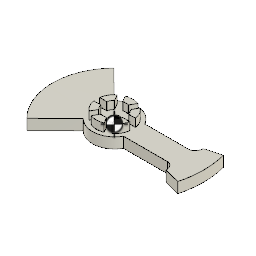
Hammer v2 v7 (Autodesk Fusion 360 design; units mm, degrees)
Autodesk Fusion 360 part; units mm, degrees
sketch "Sketch1" plane through (0, 0, 0) normal (0, 0, 1) x (1, 0, 0)
  circle A0 centre (0, 0) radius 2.7
  circle A1 centre (0, 0) radius 50
  line L0 (0, 0) -> (50, 0) construction
  line L1 (0, -6) -> (49.6387, -6)
  line L2 (0, 0) -> (48.3169, -12.864)
  spline S0 degree 5 poles (39.3956, -10.4888) (39.4086, -10.3289) (39.4175, -10.0126) (39.3796, -9.5486) (39.2342, -8.9536) (38.9326, -8.2648) (38.5571, -7.6509) (38.1484, -7.1313) (37.7328, -6.7198) (37.3076, -6.4144) (36.8464, -6.2013) (36.4204, -6.091) (36.0539, -6.0356) (35.7867, -6.01) (35.6473, -6) knots 0 0 0 0 0 0 0.1 0.2 0.3 0.4 0.5 0.6 0.7 0.8 0.9 1 1 1 1 1 1
  spline S1 degree 5 poles (39.3956, 10.4888) (39.4086, 10.3289) (39.4175, 10.0126) (39.3796, 9.5486) (39.2342, 8.9536) (38.9326, 8.2648) (38.5571, 7.6509) (38.1484, 7.1313) (37.7328, 6.7198) (37.3076, 6.4144) (36.8464, 6.2013) (36.4204, 6.091) (36.0539, 6.0356) (35.7867, 6.01) (35.6473, 6) knots 0 0 0 0 0 0 0.1 0.2 0.3 0.4 0.5 0.6 0.7 0.8 0.9 1 1 1 1 1 1
  line L3 (39.3383, -11.1958) -> (39.453, -9.7818)
  line L4 (36.4525, -6.0578) -> (34.8422, -5.9422)
  line L5 (39.3383, 11.1958) -> (39.453, 9.7818)
  line L6 (36.4525, 6.0578) -> (34.8422, 5.9422)
  line L7 (0, 0) -> (48.3169, 12.864)
  line L8 (0, 6) -> (49.6387, 6)
  circle A2 centre (0, 0) radius 35
  line L9 (0, 0) -> (-24.9638, 24.5318)
  line L10 (0, 0) -> (-24.9638, -24.5318)
  circle A3 centre (0, 0) radius 12.5
  point P0 (38, -7)
  point P1 (38, 7)
  dimension "d1" = 5.4
  dimension "d2" = 100
  dimension "d3" = 6
  dimension "d5" = 135.5
  dimension "d8" = 25
  constraint coincident A0.centre A1.centre
  constraint coincident A1 L0.end
  constraint horizontal L0
  constraint coincident A1 L1.end
  constraint horizontal L1
  constraint coincident A1 L2.end
  constraint coincident L2 S0.start
  constraint coincident L1 S0.end
  constraint midpoint S0.start L3
  constraint midpoint S0.end L4
  constraint symmetric L0 L1.start L8.start
  constraint symmetric L0 L1.end L8.end
  constraint symmetric L0 A0.centre A1.centre
  constraint symmetric L0 L2.end L7.end
  constraint symmetric L0 S0.start S1.start
  constraint symmetric L0 P0 P1
  constraint symmetric L0 S0.end S1.end
  constraint symmetric L0 L3.start L5.start
  constraint symmetric L0 L3.end L5.end
  constraint symmetric L0 L4.start L6.start
  constraint symmetric L0 L4.end L6.end
  constraint concentric A0 A2
  constraint coincident A2 L9.end
  constraint symmetric L0 L9.end L10.end
  constraint concentric A1 A3
  measures "d1" diameter of A0
  measures "d2" diameter of A1
  measures "d3" distance of L0 L1
  measures "d5" angle of L0 L9
  measures "d8" diameter of A3
extrude "Extrude1" add sketch "Sketch1" along normal mid plane 6 contours A0 L2 L7 A3 | A0 L7 L9 A3 | A0 L2 L10 A3 | A0 L9 L10 A3 | L7 L8 A3 | L1 L2 L7 L8 A2 A3 | L1 L2 A3 | A2 L9 L10 A3 | A1 L1 L8 A2 | A1 S1 L7 L8 | A1 L1 L2 S0
sketch "Sketch2" plane through (0, 0, 3) normal (0, 0, 1) x (-1, 0, 0)
  circle A0 centre (0, 0) radius 2.7
  arc A1 (8.9156, 8.7614) -> (-10.9659, 6) centre (0, 0) ccw
  line L0 (-10.9659, 6) -> (-35.6473, 6)
  spline S0 degree 5 poles (-35.6473, 6) (-35.7867, 6.01) (-36.0539, 6.0356) (-36.4204, 6.091) (-36.8464, 6.2013) (-37.3076, 6.4144) (-37.7328, 6.7198) (-38.1484, 7.1313) (-38.5571, 7.6509) (-38.9326, 8.2648) (-39.2342, 8.9536) (-39.3796, 9.5486) (-39.4175, 10.0126) (-39.4086, 10.3289) (-39.3956, 10.4888) knots -1 -1 -1 -1 -1 -1 -0.9 -0.8 -0.7 -0.6 -0.5 -0.4 -0.3 -0.2 -0.1 0 0 0 0 0 0
  line L1 (-39.3956, 10.4888) -> (-48.3169, 12.864)
  arc A2 (-48.3169, 12.864) -> (-48.3169, -12.864) centre (0, 0) ccw
  line L2 (-48.3169, -12.864) -> (-39.3956, -10.4888)
  spline S1 degree 5 poles (-39.3956, -10.4888) (-39.4086, -10.3289) (-39.4175, -10.0126) (-39.3796, -9.5486) (-39.2342, -8.9536) (-38.9326, -8.2648) (-38.5571, -7.6509) (-38.1484, -7.1313) (-37.7328, -6.7198) (-37.3076, -6.4144) (-36.8464, -6.2013) (-36.4204, -6.091) (-36.0539, -6.0356) (-35.7867, -6.01) (-35.6473, -6) knots 0 0 0 0 0 0 0.1 0.2 0.3 0.4 0.5 0.6 0.7 0.8 0.9 1 1 1 1 1 1
  line L3 (-35.6473, -6) -> (-10.9659, -6)
  arc A3 (-10.9659, -6) -> (8.9156, -8.7614) centre (0, 0) ccw
  line L4 (8.9156, -8.7614) -> (24.9638, -24.5318)
  arc A4 (24.9638, -24.5318) -> (24.9638, 24.5318) centre (0, 0) ccw
  line L5 (24.9638, 24.5318) -> (8.9156, 8.7614)
  circle A5 centre (0, 0) radius 6.1545
  circle A6 centre (0, 0) radius 10.2495
  line L6 (0, 1.65) -> (10.1158, 1.65)
  line L7 (-6.8576, -8.5778) -> (-4.5496, -4.5801)
  spline S2 degree 3 poles (-6.8799, -8.583) (-6.8781, -8.5842) (-6.876, -8.585) (-6.874, -8.5853) (-6.8719, -8.5857) (-6.8702, -8.5857) (-6.8684, -8.5854) (-6.8665, -8.585) (-6.8649, -8.5844) (-6.8634, -8.5835) (-6.8623, -8.5829) (-6.8613, -8.5822) (-6.8604, -8.5813) (-6.8593, -8.5803) (-6.8584, -8.5791) (-6.8576, -8.5778) knots -0.146478 -0.146478 -0.146478 -0.146478 -0.128978 -0.128978 -0.128978 -0.112667 -0.112667 -0.112667 -0.096104 -0.096104 -0.096104 -0.084227 -0.084227 -0.084227 -0.069674 -0.069674 -0.069674 -0.069674
  arc A7 (3.9931, 10.2496) -> (-3.9931, 10.2496) centre (0, 0) ccw
  circle A8 centre (0, 0) radius 6.335
  arc A9 (-3.9931, -10.2496) -> (3.9931, -10.2496) centre (0, 0) ccw
  circle A10 centre (0, 0) radius 16.7005
  circle A11 centre (0, 0) radius 2.7005
  spline S3 degree 3 poles (-4.3462, -10.0278) (-4.349, -10.0327) (-4.3517, -10.0376) (-4.357, -10.0477) (-4.3595, -10.0528) (-4.3635, -10.0611) (-4.3649, -10.0643) (-4.3677, -10.0705) (-4.3689, -10.0734) (-4.3717, -10.0801) (-4.3732, -10.0838) (-4.3775, -10.0951) (-4.3801, -10.1027) (-4.3954, -10.1509) (-4.402, -10.1935) (-4.4018, -10.2542) (-4.4007, -10.2718) (-4.3915, -10.3419) (-4.3744, -10.3946) (-4.3231, -10.4833) (-4.2929, -10.5203) (-4.2227, -10.5801) (-4.185, -10.6033) (-4.1437, -10.6203) knots -0.079764 -0.079764 -0.079764 -0.079764 -0.077736 -0.077736 -0.075667 -0.075667 -0.074396 -0.074396 -0.073245 -0.073245 -0.071774 -0.071774 -0.068877 -0.068877 -0.053423 -0.053423 -0.047168 -0.047168 -0.028481 -0.028481 -0.013393 -0.013393 0 0 0 0
  spline S4 degree 3 poles (-10.8574, -1.65) (-10.8584, -1.65) (-10.8595, -1.6501) (-10.8605, -1.6503) (-10.862, -1.6506) (-10.8635, -1.6511) (-10.8648, -1.6519) (-10.8666, -1.6528) (-10.8681, -1.654) (-10.8696, -1.6558) (-10.8707, -1.6572) (-10.8716, -1.6587) (-10.8722, -1.6607) (-10.8729, -1.6626) (-10.8731, -1.6646) (-10.873, -1.6667) knots -0.08749 -0.08749 -0.08749 -0.08749 -0.077534 -0.077534 -0.077534 -0.062667 -0.062667 -0.062667 -0.04351 -0.04351 -0.04351 -0.027229 -0.027229 -0.027229 -0.010666 -0.010666 -0.010666 -0.010666
  arc A12 (-11.2693, -1.7216) -> (-7.1256, -8.8987) centre (0, 0) ccw
  arc A13 (-10.873, -1.6667) -> (-6.8799, -8.583) centre (0, 0) ccw
  line L8 (-6.2412, -1.65) -> (-10.8574, -1.65)
  arc A14 (-4.2907, -4.1005) -> (-1.4057, -5.7661) centre (0, 0) ccw
  spline S5 degree 3 poles (-7.1256, -8.8987) (-7.1226, -8.9009) (-7.1197, -8.9032) (-7.0927, -8.9229) (-7.0671, -8.9377) (-6.9958, -8.9695) (-6.9495, -8.9807) (-6.8523, -8.9884) (-6.8024, -8.9827) (-6.7014, -8.9536) (-6.6517, -8.9271) (-6.5946, -8.8808) (-6.5808, -8.8679) (-6.5618, -8.8477) (-6.5559, -8.8409) (-6.5471, -8.8302) (-6.544, -8.8263) (-6.5385, -8.8191) (-6.536, -8.8158) (-6.5307, -8.8084) (-6.5279, -8.8043) (-6.5203, -8.7929) (-6.5156, -8.7854) (-6.5112, -8.7778) knots -0.080264 -0.080264 -0.080264 -0.080264 -0.079146 -0.079146 -0.070166 -0.070166 -0.055156 -0.055156 -0.03834 -0.03834 -0.018441 -0.018441 -0.011572 -0.011572 -0.008302 -0.008302 -0.006499 -0.006499 -0.004985 -0.004985 -0.003198 -0.003198 0 0 0 0
  spline S6 degree 3 poles (-6.0804, -1.7779) (-6.0844, -1.7641) (-6.0901, -1.7508) (-6.0974, -1.7384) (-6.1052, -1.7248) (-6.1149, -1.7124) (-6.126, -1.7014) (-6.1396, -1.6879) (-6.1553, -1.6766) (-6.1725, -1.6681) (-6.1877, -1.6607) (-6.2038, -1.6554) (-6.2204, -1.6524) (-6.2273, -1.6512) (-6.2343, -1.6504) (-6.2412, -1.65) knots -0.077702 -0.077702 -0.077702 -0.077702 -0.063693 -0.063693 -0.063693 -0.048454 -0.048454 -0.048454 -0.029774 -0.029774 -0.029774 -0.013339 -0.013339 -0.013339 -0.006509 -0.006509 -0.006509 -0.006509
  spline S7 degree 3 poles (-5.6965, -1.6656) (-5.7165, -1.5973) (-5.7489, -1.5333) (-5.8314, -1.4253) (-5.8791, -1.3808) (-5.9816, -1.3132) (-6.0346, -1.2888) (-6.1368, -1.2591) (-6.1847, -1.2515) (-6.2331, -1.25) knots -0.072712 -0.072712 -0.072712 -0.072712 -0.051359 -0.051359 -0.031933 -0.031933 -0.014516 -0.014516 0 0 0 0
  line L9 (-6.5112, -8.7778) -> (-4.1991, -4.773)
  arc A15 (-4.1437, -10.6203) -> (4.1437, -10.6203) centre (0, 0) ccw
  spline S8 degree 3 poles (-1.5005, -6.1547) (-1.5145, -6.1513) (-1.5288, -6.1496) (-1.5432, -6.1497) (-1.5589, -6.1497) (-1.5744, -6.1518) (-1.5895, -6.1559) (-1.6081, -6.161) (-1.6256, -6.169) (-1.6416, -6.1796) (-1.6557, -6.189) (-1.6683, -6.2003) (-1.6791, -6.2132) (-1.6837, -6.2186) (-1.6878, -6.2242) (-1.6917, -6.2301) knots -0.077702 -0.077702 -0.077702 -0.077702 -0.063693 -0.063693 -0.063693 -0.048454 -0.048454 -0.048454 -0.029774 -0.029774 -0.029774 -0.013339 -0.013339 -0.013339 -0.006509 -0.006509 -0.006509 -0.006509
  line L10 (-2.034, -6.023) -> (-4.3462, -10.0278)
  spline S9 degree 3 poles (-3.9998, -10.2278) (-4.0003, -10.2287) (-4.0007, -10.2296) (-4.001, -10.2306) (-4.0015, -10.2321) (-4.0018, -10.2336) (-4.0018, -10.2352) (-4.0019, -10.2372) (-4.0016, -10.2391) (-4.0008, -10.2412) (-4.0002, -10.2429) (-3.9993, -10.2444) (-3.9979, -10.246) (-3.9966, -10.2475) (-3.995, -10.2487) (-3.9931, -10.2496) knots -0.08749 -0.08749 -0.08749 -0.08749 -0.077534 -0.077534 -0.077534 -0.062667 -0.062667 -0.062667 -0.04351 -0.04351 -0.04351 -0.027229 -0.027229 -0.027229 -0.010666 -0.010666 -0.010666 -0.010666
  line L11 (-1.6917, -6.2301) -> (-3.9998, -10.2278)
  line L12 (-6.2331, -1.25) -> (-10.8574, -1.25)
  circle A16 centre (0, 0) radius 5.935
  spline S10 degree 3 poles (-4.1437, 10.6203) (-4.1757, 10.6071) (-4.2057, 10.5902) (-4.2631, 10.5478) (-4.2894, 10.5222) (-4.3436, 10.4539) (-4.3668, 10.4095) (-4.3963, 10.3184) (-4.4028, 10.2717) (-4.401, 10.1948) (-4.3968, 10.164) (-4.386, 10.1213) (-4.3822, 10.1087) (-4.376, 10.0912) (-4.3741, 10.0862) (-4.3709, 10.0781) (-4.3696, 10.0749) (-4.3669, 10.0688) (-4.3656, 10.0659) (-4.3626, 10.0592) (-4.3608, 10.0554) (-4.3551, 10.0438) (-4.3509, 10.0361) (-4.3464, 10.0282) (-4.3463, 10.028) (-4.3462, 10.0278) knots -0.099601 -0.099601 -0.099601 -0.099601 -0.089178 -0.089178 -0.077713 -0.077713 -0.061196 -0.061196 -0.044718 -0.044718 -0.033484 -0.033484 -0.028686 -0.028686 -0.026742 -0.026742 -0.025496 -0.025496 -0.024331 -0.024331 -0.022814 -0.022814 -0.019643 -0.019643 -0.019544 -0.019544 -0.019544 -0.019544
  line L13 (-10.8574, 1.65) -> (-6.2412, 1.65)
  spline S11 degree 3 poles (-6.8576, 8.5778) (-6.8582, 8.5787) (-6.8588, 8.5795) (-6.8594, 8.5803) (-6.8605, 8.5815) (-6.8617, 8.5825) (-6.863, 8.5833) (-6.8647, 8.5843) (-6.8665, 8.5851) (-6.8687, 8.5854) (-6.8705, 8.5857) (-6.8723, 8.5857) (-6.8743, 8.5853) (-6.8763, 8.5849) (-6.8782, 8.5841) (-6.8799, 8.583) knots -0.08749 -0.08749 -0.08749 -0.08749 -0.077534 -0.077534 -0.077534 -0.062667 -0.062667 -0.062667 -0.04351 -0.04351 -0.04351 -0.027229 -0.027229 -0.027229 -0.010666 -0.010666 -0.010666 -0.010666
  spline S12 degree 3 poles (-2.034, 6.023) (-1.9994, 5.9673) (-1.9556, 5.9178) (-1.8735, 5.852) (-1.84, 5.8304) (-1.7506, 5.7849) (-1.6926, 5.7661) (-1.5572, 5.7448) (-1.48, 5.748) (-1.4057, 5.7661) knots -0.072724 -0.072724 -0.072724 -0.072724 -0.053033 -0.053033 -0.041123 -0.041123 -0.02294 -0.02294 0 0 0 0
  line L14 (-4.3462, 10.0278) -> (-2.034, 6.023)
  arc A17 (-1.4057, 5.7661) -> (-4.2907, 4.1005) centre (0, 0) ccw
  spline S13 degree 3 poles (-1.6917, 6.2301) (-1.6814, 6.2144) (-1.6688, 6.2005) (-1.6542, 6.1888) (-1.6446, 6.1812) (-1.6343, 6.1745) (-1.6234, 6.169) (-1.6068, 6.1605) (-1.5889, 6.1547) (-1.5704, 6.1518) (-1.5472, 6.1482) (-1.5234, 6.1492) (-1.5005, 6.1547) knots -0.071247 -0.071247 -0.071247 -0.071247 -0.05302 -0.05302 -0.05302 -0.041116 -0.041116 -0.041116 -0.022939 -0.022939 -0.022939 0 0 0 0
  line L15 (-3.9998, 10.2278) -> (-1.6917, 6.2301)
  spline S14 degree 3 poles (-4.5496, -4.5801) (-4.5412, -4.5634) (-4.5354, -4.5455) (-4.5326, -4.527) (-4.5307, -4.5149) (-4.5301, -4.5026) (-4.5308, -4.4904) (-4.5318, -4.4718) (-4.5357, -4.4534) (-4.5424, -4.436) (-4.5509, -4.414) (-4.5636, -4.3939) (-4.5799, -4.3768) knots -0.071247 -0.071247 -0.071247 -0.071247 -0.05302 -0.05302 -0.05302 -0.041116 -0.041116 -0.041116 -0.022939 -0.022939 -0.022939 0 0 0 0
  spline S15 degree 3 poles (-6.2412, 1.65) (-6.2226, 1.6511) (-6.2042, 1.6551) (-6.1868, 1.6619) (-6.1754, 1.6663) (-6.1645, 1.6719) (-6.1542, 1.6786) (-6.1386, 1.6888) (-6.1246, 1.7014) (-6.1129, 1.7159) (-6.0981, 1.7342) (-6.087, 1.7553) (-6.0804, 1.7779) knots -0.071247 -0.071247 -0.071247 -0.071247 -0.05302 -0.05302 -0.05302 -0.041116 -0.041116 -0.041116 -0.022939 -0.022939 -0.022939 0 0 0 0
  spline S16 degree 3 poles (-10.8574, -1.25) (-10.8623, -1.25) (-10.8672, -1.2501) (-10.8783, -1.2505) (-10.8845, -1.2508) (-10.8945, -1.2516) (-10.8984, -1.252) (-10.9058, -1.2528) (-10.9094, -1.2532) (-10.9175, -1.2543) (-10.9221, -1.255) (-10.9363, -1.2574) (-10.9458, -1.2594) (-11.0105, -1.2751) (-11.063, -1.2998) (-11.1532, -1.3685) (-11.1916, -1.4115) (-11.2435, -1.5046) (-11.2601, -1.5511) (-11.2742, -1.6405) (-11.2748, -1.6811) (-11.2693, -1.7216) knots -0.086203 -0.086203 -0.086203 -0.086203 -0.084433 -0.084433 -0.082213 -0.082213 -0.08081 -0.08081 -0.079512 -0.079512 -0.077841 -0.077841 -0.0743 -0.0743 -0.053753 -0.053753 -0.034336 -0.034336 -0.018768 -0.018768 -0.006485 -0.006485 -0.006485 -0.006485
  arc A18 (-7.1256, 8.8987) -> (-11.2693, 1.7216) centre (0, 0) ccw
  spline S17 degree 3 poles (-1.4057, -5.7661) (-1.4298, -5.7603) (-1.4542, -5.7559) (-1.5247, -5.7481) (-1.571, -5.7485) (-1.681, -5.7627) (-1.7434, -5.7818) (-1.8533, -5.8367) (-1.901, -5.8704) (-1.9779, -5.9441) (-2.0085, -5.9819) (-2.034, -6.023) knots -0.072677 -0.072677 -0.072677 -0.072677 -0.065242 -0.065242 -0.051396 -0.051396 -0.031964 -0.031964 -0.014535 -0.014535 0 0 0 0
  line L16 (-4.5496, 4.5801) -> (-6.8576, 8.5778)
  spline S18 degree 3 poles (-11.2693, 1.7216) (-11.272, 1.7015) (-11.2732, 1.6813) (-11.2725, 1.6136) (-11.2639, 1.5679) (-11.2314, 1.4771) (-11.2059, 1.4341) (-11.1436, 1.3604) (-11.1068, 1.3299) (-11.0381, 1.2899) (-11.0078, 1.2768) (-10.9639, 1.2637) (-10.9512, 1.2605) (-10.9321, 1.2567) (-10.9258, 1.2556) (-10.9155, 1.2541) (-10.9116, 1.2535) (-10.9042, 1.2526) (-10.9006, 1.2522) (-10.8925, 1.2515) (-10.8879, 1.2511) (-10.8747, 1.2503) (-10.8661, 1.25) (-10.8574, 1.25) knots -0.149421 -0.149421 -0.149421 -0.149421 -0.143292 -0.143292 -0.128978 -0.128978 -0.112667 -0.112667 -0.096104 -0.096104 -0.084227 -0.084227 -0.079495 -0.079495 -0.07717 -0.07717 -0.075742 -0.075742 -0.074448 -0.074448 -0.072794 -0.072794 -0.069674 -0.069674 -0.069674 -0.069674
  spline S19 degree 3 poles (-4.1991, -4.773) (-4.1836, -4.7441) (-4.1705, -4.7138) (-4.1512, -4.6556) (-4.1442, -4.628) (-4.132, -4.5588) (-4.1293, -4.517) (-4.1337, -4.4126) (-4.1466, -4.3508) (-4.1966, -4.221) (-4.2379, -4.1557) (-4.2907, -4.1005) knots -0.072701 -0.072701 -0.072701 -0.072701 -0.062829 -0.062829 -0.054287 -0.054287 -0.041746 -0.041746 -0.02294 -0.02294 0 0 0 0
  line L17 (-4.1991, 4.773) -> (-6.5112, 8.7778)
  spline S20 degree 3 poles (-10.873, 1.6667) (-10.8731, 1.6645) (-10.8728, 1.6623) (-10.8721, 1.6604) (-10.8714, 1.6584) (-10.8705, 1.6569) (-10.8693, 1.6556) (-10.8681, 1.6541) (-10.8668, 1.653) (-10.8653, 1.6521) (-10.8642, 1.6515) (-10.863, 1.651) (-10.8619, 1.6507) (-10.8604, 1.6502) (-10.8589, 1.65) (-10.8574, 1.65) knots -0.146478 -0.146478 -0.146478 -0.146478 -0.128978 -0.128978 -0.128978 -0.112667 -0.112667 -0.112667 -0.096104 -0.096104 -0.096104 -0.084227 -0.084227 -0.084227 -0.069674 -0.069674 -0.069674 -0.069674
  arc A19 (4.1437, 10.6203) -> (-4.1437, 10.6203) centre (0, 0) ccw
  spline S21 degree 3 poles (-3.9931, 10.2496) (-3.9951, 10.2487) (-3.9968, 10.2473) (-3.9981, 10.2457) (-3.9995, 10.2441) (-4.0003, 10.2426) (-4.0009, 10.2409) (-4.0016, 10.2391) (-4.0018, 10.2374) (-4.0018, 10.2357) (-4.0019, 10.2344) (-4.0017, 10.2332) (-4.0014, 10.232) (-4.0011, 10.2305) (-4.0005, 10.2291) (-3.9998, 10.2278) knots -0.146478 -0.146478 -0.146478 -0.146478 -0.128978 -0.128978 -0.128978 -0.112667 -0.112667 -0.112667 -0.096104 -0.096104 -0.096104 -0.084227 -0.084227 -0.084227 -0.069674 -0.069674 -0.069674 -0.069674
  arc A20 (-6.8799, 8.583) -> (-10.873, 1.6667) centre (0, 0) ccw
  spline S22 degree 3 poles (-4.2907, 4.1005) (-4.2585, 4.1342) (-4.2304, 4.1718) (-4.1819, 4.2563) (-4.1626, 4.3035) (-4.1338, 4.4129) (-4.1277, 4.4752) (-4.1353, 4.592) (-4.1466, 4.6459) (-4.1747, 4.7234) (-4.186, 4.7486) (-4.1991, 4.773) knots -0.077702 -0.077702 -0.077702 -0.077702 -0.063693 -0.063693 -0.048454 -0.048454 -0.029774 -0.029774 -0.013339 -0.013339 -0.00503 -0.00503 -0.00503 -0.00503
  circle A21 centre (0, 0) radius 13.9
  spline S23 degree 3 poles (-4.5799, 4.3768) (-4.57, 4.3872) (-4.5613, 4.3988) (-4.5542, 4.4113) (-4.5464, 4.4249) (-4.5404, 4.4394) (-4.5364, 4.4546) (-4.5315, 4.4731) (-4.5297, 4.4923) (-4.5309, 4.5115) (-4.532, 4.5283) (-4.5355, 4.5449) (-4.5412, 4.5608) (-4.5436, 4.5674) (-4.5464, 4.5738) (-4.5496, 4.5801) knots -0.077702 -0.077702 -0.077702 -0.077702 -0.063693 -0.063693 -0.063693 -0.048454 -0.048454 -0.048454 -0.029774 -0.029774 -0.029774 -0.013339 -0.013339 -0.013339 -0.006509 -0.006509 -0.006509 -0.006509
  spline S24 degree 3 poles (-6.5112, 8.7778) (-6.5152, 8.7846) (-6.5193, 8.7914) (-6.526, 8.8015) (-6.5283, 8.8049) (-6.5332, 8.8119) (-6.5356, 8.8153) (-6.5409, 8.8223) (-6.5436, 8.8258) (-6.5506, 8.8345) (-6.5549, 8.8397) (-6.571, 8.858) (-6.5835, 8.8704) (-6.6143, 8.8975) (-6.6332, 8.9116) (-6.6989, 8.952) (-6.7506, 8.9717) (-6.8537, 8.988) (-6.9038, 8.9875) (-6.9977, 8.9684) (-7.0406, 8.9524) (-7.0964, 8.9198) (-7.1114, 8.9097) (-7.1256, 8.8987) knots -0.08749 -0.08749 -0.08749 -0.08749 -0.084639 -0.084639 -0.083129 -0.083129 -0.081593 -0.081593 -0.079982 -0.079982 -0.077534 -0.077534 -0.071156 -0.071156 -0.062667 -0.062667 -0.04351 -0.04351 -0.027229 -0.027229 -0.013166 -0.013166 -0.007722 -0.007722 -0.007722 -0.007722
  spline S25 degree 3 poles (-6.2331, 1.25) (-6.1675, 1.2521) (-6.1027, 1.2653) (-6.0046, 1.3036) (-5.9692, 1.3217) (-5.8852, 1.3764) (-5.8399, 1.4173) (-5.7537, 1.5238) (-5.7179, 1.5923) (-5.6965, 1.6656) knots -0.072724 -0.072724 -0.072724 -0.072724 -0.05302 -0.05302 -0.041116 -0.041116 -0.022939 -0.022939 0 0 0 0
  spline S26 degree 3 poles (1.6917, -6.2301) (1.6814, -6.2144) (1.6688, -6.2005) (1.6542, -6.1888) (1.6446, -6.1812) (1.6343, -6.1745) (1.6234, -6.169) (1.6068, -6.1605) (1.5889, -6.1547) (1.5704, -6.1518) (1.5472, -6.1482) (1.5234, -6.1492) (1.5005, -6.1547) knots -0.071247 -0.071247 -0.071247 -0.071247 -0.05302 -0.05302 -0.05302 -0.041116 -0.041116 -0.041116 -0.022939 -0.022939 -0.022939 0 0 0 0
  spline S27 degree 3 poles (10.873, -1.6667) (10.8731, -1.6645) (10.8728, -1.6623) (10.8721, -1.6604) (10.8714, -1.6584) (10.8705, -1.6569) (10.8693, -1.6556) (10.8681, -1.6541) (10.8668, -1.653) (10.8653, -1.6521) (10.8642, -1.6515) (10.863, -1.651) (10.8619, -1.6507) (10.8604, -1.6502) (10.8589, -1.65) (10.8574, -1.65) knots -0.146478 -0.146478 -0.146478 -0.146478 -0.128978 -0.128978 -0.128978 -0.112667 -0.112667 -0.112667 -0.096104 -0.096104 -0.096104 -0.084227 -0.084227 -0.084227 -0.069674 -0.069674 -0.069674 -0.069674
  spline S28 degree 3 poles (2.034, -6.023) (1.9994, -5.9673) (1.9556, -5.9178) (1.8735, -5.852) (1.84, -5.8304) (1.7506, -5.7849) (1.6926, -5.7661) (1.5572, -5.7448) (1.48, -5.748) (1.4057, -5.7661) knots -0.072724 -0.072724 -0.072724 -0.072724 -0.053033 -0.053033 -0.041123 -0.041123 -0.02294 -0.02294 0 0 0 0
  line L18 (-10.8574, 1.25) -> (-6.2331, 1.25)
  spline S29 degree 3 poles (6.2412, -1.65) (6.2226, -1.6511) (6.2042, -1.6551) (6.1868, -1.6619) (6.1754, -1.6663) (6.1645, -1.6719) (6.1542, -1.6786) (6.1386, -1.6888) (6.1246, -1.7014) (6.1129, -1.7159) (6.0981, -1.7342) (6.087, -1.7553) (6.0804, -1.7779) knots -0.071247 -0.071247 -0.071247 -0.071247 -0.05302 -0.05302 -0.05302 -0.041116 -0.041116 -0.041116 -0.022939 -0.022939 -0.022939 0 0 0 0
  spline S30 degree 3 poles (6.2331, -1.25) (6.1675, -1.2521) (6.1027, -1.2653) (6.0046, -1.3036) (5.9692, -1.3217) (5.8852, -1.3764) (5.8399, -1.4173) (5.7537, -1.5238) (5.7179, -1.5923) (5.6965, -1.6656) knots -0.072724 -0.072724 -0.072724 -0.072724 -0.05302 -0.05302 -0.041116 -0.041116 -0.022939 -0.022939 0 0 0 0
  line L19 (4.5496, -4.5801) -> (6.8576, -8.5778)
  line L20 (4.3462, -10.0278) -> (2.034, -6.023)
  arc A22 (7.1256, -8.8987) -> (11.2693, -1.7216) centre (0, 0) ccw
  spline S31 degree 3 poles (6.8576, -8.5778) (6.8582, -8.5787) (6.8588, -8.5795) (6.8594, -8.5803) (6.8605, -8.5815) (6.8617, -8.5825) (6.863, -8.5833) (6.8647, -8.5843) (6.8665, -8.5851) (6.8687, -8.5854) (6.8705, -8.5857) (6.8723, -8.5857) (6.8743, -8.5853) (6.8763, -8.5849) (6.8782, -8.5841) (6.8799, -8.583) knots -0.08749 -0.08749 -0.08749 -0.08749 -0.077534 -0.077534 -0.077534 -0.062667 -0.062667 -0.062667 -0.04351 -0.04351 -0.04351 -0.027229 -0.027229 -0.027229 -0.010666 -0.010666 -0.010666 -0.010666
  arc A23 (-5.6965, 1.6656) -> (-5.6965, -1.6656) centre (0, 0) ccw
  spline S32 degree 3 poles (3.9931, -10.2496) (3.9951, -10.2487) (3.9968, -10.2473) (3.9981, -10.2457) (3.9995, -10.2441) (4.0003, -10.2426) (4.0009, -10.2409) (4.0016, -10.2391) (4.0018, -10.2374) (4.0018, -10.2357) (4.0019, -10.2344) (4.0017, -10.2332) (4.0014, -10.232) (4.0011, -10.2305) (4.0005, -10.2291) (3.9998, -10.2278) knots -0.146478 -0.146478 -0.146478 -0.146478 -0.128978 -0.128978 -0.128978 -0.112667 -0.112667 -0.112667 -0.096104 -0.096104 -0.096104 -0.084227 -0.084227 -0.084227 -0.069674 -0.069674 -0.069674 -0.069674
  spline S33 degree 3 poles (11.2693, -1.7216) (11.272, -1.7015) (11.2732, -1.6813) (11.2725, -1.6136) (11.2639, -1.5679) (11.2314, -1.4771) (11.2059, -1.4341) (11.1436, -1.3604) (11.1068, -1.3299) (11.0381, -1.2899) (11.0078, -1.2768) (10.9639, -1.2637) (10.9512, -1.2605) (10.9321, -1.2567) (10.9258, -1.2556) (10.9155, -1.2541) (10.9116, -1.2535) (10.9042, -1.2526) (10.9006, -1.2522) (10.8925, -1.2515) (10.8879, -1.2511) (10.8747, -1.2503) (10.8661, -1.25) (10.8574, -1.25) knots -0.149421 -0.149421 -0.149421 -0.149421 -0.143292 -0.143292 -0.128978 -0.128978 -0.112667 -0.112667 -0.096104 -0.096104 -0.084227 -0.084227 -0.079495 -0.079495 -0.07717 -0.07717 -0.075742 -0.075742 -0.074448 -0.074448 -0.072794 -0.072794 -0.069674 -0.069674 -0.069674 -0.069674
  arc A24 (1.4057, -5.7661) -> (4.2907, -4.1005) centre (0, 0) ccw
  spline S34 degree 3 poles (4.5799, -4.3768) (4.57, -4.3872) (4.5613, -4.3988) (4.5542, -4.4113) (4.5464, -4.4249) (4.5404, -4.4394) (4.5364, -4.4546) (4.5315, -4.4731) (4.5297, -4.4923) (4.5309, -4.5115) (4.532, -4.5283) (4.5355, -4.5449) (4.5412, -4.5608) (4.5436, -4.5674) (4.5464, -4.5738) (4.5496, -4.5801) knots -0.077702 -0.077702 -0.077702 -0.077702 -0.063693 -0.063693 -0.063693 -0.048454 -0.048454 -0.048454 -0.029774 -0.029774 -0.029774 -0.013339 -0.013339 -0.013339 -0.006509 -0.006509 -0.006509 -0.006509
  spline S35 degree 3 poles (7.1256, 8.8987) (7.1226, 8.9009) (7.1197, 8.9032) (7.0927, 8.9229) (7.0671, 8.9377) (6.9958, 8.9695) (6.9495, 8.9807) (6.8523, 8.9884) (6.8024, 8.9827) (6.7014, 8.9536) (6.6517, 8.9271) (6.5946, 8.8808) (6.5808, 8.8679) (6.5618, 8.8477) (6.5559, 8.8409) (6.5471, 8.8302) (6.544, 8.8263) (6.5385, 8.8191) (6.536, 8.8158) (6.5307, 8.8084) (6.5279, 8.8043) (6.5203, 8.7929) (6.5156, 8.7854) (6.5112, 8.7778) knots -0.080264 -0.080264 -0.080264 -0.080264 -0.079146 -0.079146 -0.070166 -0.070166 -0.055156 -0.055156 -0.03834 -0.03834 -0.018441 -0.018441 -0.011572 -0.011572 -0.008302 -0.008302 -0.006499 -0.006499 -0.004985 -0.004985 -0.003198 -0.003198 0 0 0 0
  spline S36 degree 3 poles (5.6965, 1.6656) (5.7165, 1.5973) (5.7489, 1.5333) (5.8314, 1.4253) (5.8791, 1.3808) (5.9816, 1.3132) (6.0346, 1.2888) (6.1368, 1.2591) (6.1847, 1.2515) (6.2331, 1.25) knots -0.072712 -0.072712 -0.072712 -0.072712 -0.051359 -0.051359 -0.031933 -0.031933 -0.014516 -0.014516 0 0 0 0
  spline S37 degree 3 poles (4.1437, -10.6203) (4.1757, -10.6071) (4.2057, -10.5902) (4.2631, -10.5478) (4.2894, -10.5222) (4.3436, -10.4539) (4.3668, -10.4095) (4.3963, -10.3184) (4.4028, -10.2717) (4.401, -10.1948) (4.3968, -10.164) (4.386, -10.1213) (4.3822, -10.1087) (4.376, -10.0912) (4.3741, -10.0862) (4.3709, -10.0781) (4.3696, -10.0749) (4.3669, -10.0688) (4.3656, -10.0659) (4.3626, -10.0592) (4.3608, -10.0554) (4.3551, -10.0438) (4.3509, -10.0361) (4.3464, -10.0282) (4.3463, -10.028) (4.3462, -10.0278) knots -0.099601 -0.099601 -0.099601 -0.099601 -0.089178 -0.089178 -0.077713 -0.077713 -0.061196 -0.061196 -0.044718 -0.044718 -0.033484 -0.033484 -0.028686 -0.028686 -0.026742 -0.026742 -0.025496 -0.025496 -0.024331 -0.024331 -0.022814 -0.022814 -0.019643 -0.019643 -0.019544 -0.019544 -0.019544 -0.019544
  spline S38 degree 3 poles (1.4057, 5.7661) (1.4748, 5.7493) (1.5463, 5.7453) (1.681, 5.7627) (1.7434, 5.7818) (1.8533, 5.8367) (1.901, 5.8704) (1.9779, 5.9441) (2.0085, 5.9819) (2.034, 6.023) knots -0.072711 -0.072711 -0.072711 -0.072711 -0.051396 -0.051396 -0.031964 -0.031964 -0.014535 -0.014535 0 0 0 0
  arc A25 (5.6965, -1.6656) -> (5.6965, 1.6656) centre (0, 0) ccw
  spline S39 degree 3 poles (4.3462, 10.0278) (4.349, 10.0327) (4.3517, 10.0376) (4.357, 10.0477) (4.3595, 10.0528) (4.3635, 10.0611) (4.3649, 10.0643) (4.3677, 10.0705) (4.3689, 10.0734) (4.3717, 10.0801) (4.3732, 10.0838) (4.3775, 10.0951) (4.3801, 10.1027) (4.3954, 10.1509) (4.402, 10.1935) (4.4018, 10.2542) (4.4007, 10.2718) (4.3915, 10.3419) (4.3744, 10.3946) (4.3231, 10.4833) (4.2929, 10.5203) (4.2227, 10.5801) (4.185, 10.6033) (4.1437, 10.6203) knots -0.079764 -0.079764 -0.079764 -0.079764 -0.077736 -0.077736 -0.075667 -0.075667 -0.074396 -0.074396 -0.073245 -0.073245 -0.071774 -0.071774 -0.068877 -0.068877 -0.053423 -0.053423 -0.047168 -0.047168 -0.028481 -0.028481 -0.013393 -0.013393 0 0 0 0
  line L21 (3.9998, -10.2278) -> (1.6917, -6.2301)
  line L22 (6.2331, 1.25) -> (10.8574, 1.25)
  spline S40 degree 3 poles (6.5112, -8.7778) (6.5152, -8.7846) (6.5193, -8.7914) (6.526, -8.8015) (6.5283, -8.8049) (6.5332, -8.8119) (6.5356, -8.8153) (6.5409, -8.8223) (6.5436, -8.8258) (6.5506, -8.8345) (6.5549, -8.8397) (6.571, -8.858) (6.5835, -8.8704) (6.6143, -8.8975) (6.6332, -8.9116) (6.6989, -8.952) (6.7506, -8.9717) (6.8537, -8.988) (6.9038, -8.9875) (6.9977, -8.9684) (7.0406, -8.9524) (7.0964, -8.9198) (7.1114, -8.9097) (7.1256, -8.8987) knots -0.08749 -0.08749 -0.08749 -0.08749 -0.084639 -0.084639 -0.083129 -0.083129 -0.081593 -0.081593 -0.079982 -0.079982 -0.077534 -0.077534 -0.071156 -0.071156 -0.062667 -0.062667 -0.04351 -0.04351 -0.027229 -0.027229 -0.013166 -0.013166 -0.007722 -0.007722 -0.007722 -0.007722
  line L23 (1.6917, 6.2301) -> (3.9998, 10.2278)
  spline S41 degree 3 poles (1.5005, 6.1547) (1.5145, 6.1513) (1.5288, 6.1496) (1.5432, 6.1497) (1.5589, 6.1497) (1.5744, 6.1518) (1.5895, 6.1559) (1.6081, 6.161) (1.6256, 6.169) (1.6416, 6.1796) (1.6557, 6.189) (1.6683, 6.2003) (1.6791, 6.2132) (1.6837, 6.2186) (1.6878, 6.2242) (1.6917, 6.2301) knots -0.077702 -0.077702 -0.077702 -0.077702 -0.063693 -0.063693 -0.063693 -0.048454 -0.048454 -0.048454 -0.029774 -0.029774 -0.029774 -0.013339 -0.013339 -0.013339 -0.006509 -0.006509 -0.006509 -0.006509
  spline S42 degree 3 poles (6.0804, 1.7779) (6.0844, 1.7641) (6.0901, 1.7508) (6.0974, 1.7384) (6.1052, 1.7248) (6.1149, 1.7124) (6.126, 1.7014) (6.1396, 1.6879) (6.1553, 1.6766) (6.1725, 1.6681) (6.1877, 1.6607) (6.2038, 1.6554) (6.2204, 1.6524) (6.2273, 1.6512) (6.2343, 1.6504) (6.2412, 1.65) knots -0.077702 -0.077702 -0.077702 -0.077702 -0.063693 -0.063693 -0.063693 -0.048454 -0.048454 -0.048454 -0.029774 -0.029774 -0.029774 -0.013339 -0.013339 -0.013339 -0.006509 -0.006509 -0.006509 -0.006509
  arc A26 (6.8799, -8.583) -> (10.873, -1.6667) centre (0, 0) ccw
  spline S43 degree 3 poles (4.2907, -4.1005) (4.2585, -4.1342) (4.2304, -4.1718) (4.1819, -4.2563) (4.1626, -4.3035) (4.1338, -4.4129) (4.1277, -4.4752) (4.1353, -4.592) (4.1466, -4.6459) (4.1747, -4.7234) (4.186, -4.7486) (4.1991, -4.773) knots -0.077702 -0.077702 -0.077702 -0.077702 -0.063693 -0.063693 -0.048454 -0.048454 -0.029774 -0.029774 -0.013339 -0.013339 -0.00503 -0.00503 -0.00503 -0.00503
  spline S44 degree 3 poles (6.8799, 8.583) (6.8781, 8.5842) (6.876, 8.585) (6.874, 8.5853) (6.8719, 8.5857) (6.8702, 8.5857) (6.8684, 8.5854) (6.8665, 8.585) (6.8649, 8.5844) (6.8634, 8.5835) (6.8623, 8.5829) (6.8613, 8.5822) (6.8604, 8.5813) (6.8593, 8.5803) (6.8584, 8.5791) (6.8576, 8.5778) knots -0.146478 -0.146478 -0.146478 -0.146478 -0.128978 -0.128978 -0.128978 -0.112667 -0.112667 -0.112667 -0.096104 -0.096104 -0.096104 -0.084227 -0.084227 -0.084227 -0.069674 -0.069674 -0.069674 -0.069674
  line L24 (6.8576, 8.5778) -> (4.5496, 4.5801)
  line L25 (10.8574, -1.65) -> (6.2412, -1.65)
  line L26 (4.1991, -4.773) -> (6.5112, -8.7778)
  line L27 (6.2412, 1.65) -> (10.8574, 1.65)
  spline S45 degree 3 poles (10.8574, 1.65) (10.8584, 1.65) (10.8595, 1.6501) (10.8605, 1.6503) (10.862, 1.6506) (10.8635, 1.6511) (10.8648, 1.6519) (10.8666, 1.6528) (10.8681, 1.654) (10.8696, 1.6558) (10.8707, 1.6572) (10.8716, 1.6587) (10.8722, 1.6607) (10.8729, 1.6626) (10.8731, 1.6646) (10.873, 1.6667) knots -0.08749 -0.08749 -0.08749 -0.08749 -0.077534 -0.077534 -0.077534 -0.062667 -0.062667 -0.062667 -0.04351 -0.04351 -0.04351 -0.027229 -0.027229 -0.027229 -0.010666 -0.010666 -0.010666 -0.010666
  spline S46 degree 3 poles (4.5496, 4.5801) (4.5412, 4.5634) (4.5354, 4.5455) (4.5326, 4.527) (4.5307, 4.5149) (4.5301, 4.5026) (4.5308, 4.4904) (4.5318, 4.4718) (4.5357, 4.4534) (4.5424, 4.436) (4.5509, 4.414) (4.5636, 4.3939) (4.5799, 4.3768) knots -0.071247 -0.071247 -0.071247 -0.071247 -0.05302 -0.05302 -0.05302 -0.041116 -0.041116 -0.041116 -0.022939 -0.022939 -0.022939 0 0 0 0
  arc A27 (10.873, 1.6667) -> (6.8799, 8.583) centre (0, 0) ccw
  spline S47 degree 3 poles (4.1991, 4.773) (4.1836, 4.7441) (4.1705, 4.7138) (4.1512, 4.6556) (4.1442, 4.628) (4.132, 4.5588) (4.1293, 4.517) (4.1337, 4.4126) (4.1466, 4.3508) (4.1966, 4.221) (4.2379, 4.1557) (4.2907, 4.1005) knots -0.072701 -0.072701 -0.072701 -0.072701 -0.062829 -0.062829 -0.054287 -0.054287 -0.041746 -0.041746 -0.02294 -0.02294 0 0 0 0
  arc A28 (4.2907, 4.1005) -> (1.4057, 5.7661) centre (0, 0) ccw
  line L28 (6.5112, 8.7778) -> (4.1991, 4.773)
  arc A29 (11.2693, 1.7216) -> (7.1256, 8.8987) centre (0, 0) ccw
  line L29 (2.034, 6.023) -> (4.3462, 10.0278)
  line L30 (10.8574, -1.25) -> (6.2331, -1.25)
  spline S48 degree 3 poles (3.9998, 10.2278) (4.0003, 10.2287) (4.0007, 10.2296) (4.001, 10.2306) (4.0015, 10.2321) (4.0018, 10.2336) (4.0018, 10.2352) (4.0019, 10.2372) (4.0016, 10.2391) (4.0008, 10.2412) (4.0002, 10.2429) (3.9993, 10.2444) (3.9979, 10.246) (3.9966, 10.2475) (3.995, 10.2487) (3.9931, 10.2496) knots -0.08749 -0.08749 -0.08749 -0.08749 -0.077534 -0.077534 -0.077534 -0.062667 -0.062667 -0.062667 -0.04351 -0.04351 -0.04351 -0.027229 -0.027229 -0.027229 -0.010666 -0.010666 -0.010666 -0.010666
  spline S49 degree 3 poles (10.8574, 1.25) (10.8623, 1.25) (10.8672, 1.2501) (10.8783, 1.2505) (10.8845, 1.2508) (10.8945, 1.2516) (10.8984, 1.252) (10.9058, 1.2528) (10.9094, 1.2532) (10.9175, 1.2543) (10.9221, 1.255) (10.9363, 1.2574) (10.9458, 1.2594) (11.0105, 1.2751) (11.063, 1.2998) (11.1532, 1.3685) (11.1916, 1.4115) (11.2435, 1.5046) (11.2601, 1.5511) (11.2742, 1.6405) (11.2748, 1.6811) (11.2693, 1.7216) knots -0.086203 -0.086203 -0.086203 -0.086203 -0.084433 -0.084433 -0.082213 -0.082213 -0.08081 -0.08081 -0.079512 -0.079512 -0.077841 -0.077841 -0.0743 -0.0743 -0.053753 -0.053753 -0.034336 -0.034336 -0.018768 -0.018768 -0.006485 -0.006485 -0.006485 -0.006485
  dimension "d13" = -0.4
  dimension "d17" = 360
  constraint coincident A0.centre A1.centre
  constraint concentric A16 A25
  constraint concentric A8 A16
  constraint coincident S23.start A8
extrude "Extrude2" add sketch "Sketch2" along normal blind 4.5 contours A6 A8 S29 L19 S34 L25 | A6 L6 A8 S42 L24 L27 S46 | A6 A8 S8 L11 S26 L21 | A6 A8 S13 L15 L23 S41 | A6 L7 A8 L8 S6 S14 | A6 A8 L13 S15 L16 S23
